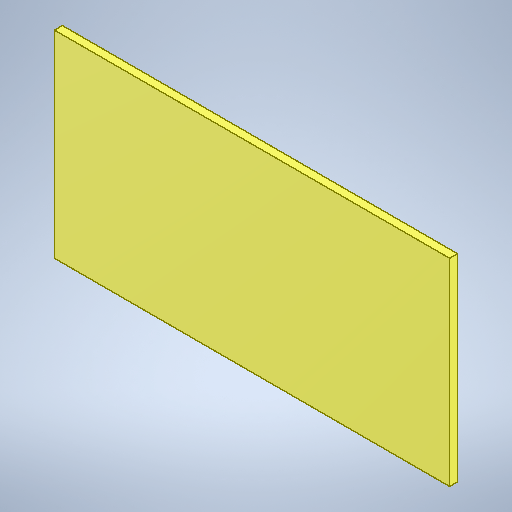
# Autodesk Inventor part: Mesa_001_0001
Saved by Autodesk Inventor 2025.2 (Build 292293000, 293)
## iProperties
Created: 2025-04-07
Part Number: Mesa_001_0001
Material: Glass
Document SubType Name: Modeling
Designer: ishad
Density: 2.18 g/cm^3
Appearance: Smooth - Yellow
Author: ishad
Autodesk Inventor part; units mm, degrees
ref_plane "YZ Plane" through (0, 0, 0) normal (1, 0, 0) x (0, 1, 0)
ref_plane "XZ Plane" through (0, 0, 0) normal (0, 1, 0) x (-1, 0, 0)
ref_plane "XY Plane" through (0, 0, 0) normal (0, 0, 1) x (1, 0, 0)
sketch "Sketch1" plane through (0, 0, 0) normal (0, 0, 1) x (1, 0, 0)
  line L0 (750, -375) -> (-750, -375)
  line L1 (-750, -375) -> (-750, 375)
  line L2 (-750, 375) -> (750, 375)
  line L3 (750, 375) -> (750, -375)
  line L4 (750, -375) -> (-750, 375) construction
  line L5 (-750, -375) -> (750, 375) construction
  point P0 (0, 0)
  dimension "d0" = 1500
  dimension "d1" = 750
  constraints: 12 end point, 2 midpoint, 2 parallel, 1 horizontal, 1 perpendicular
  measures "d0" distance of L1.end L2.end
  measures "d1" distance between parallel lines of L0 L2
extrude "Extrusion1" add sketch "Sketch1" along normal blind 30
body "Solid1"
